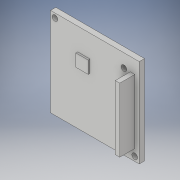
# Autodesk Inventor part: lab 04
Saved by Autodesk Inventor 2017 (Build 210142000, 142)
## iProperties
Created: 2016-10-26
Part Number: lab 04
Material: Generic
Document SubType Name: Modeling
Designer: radrajith
Density: 1 g/cm^3
Appearance: Default
Author: radrajith
Autodesk Inventor part; units mm, degrees
ref_plane "YZ Plane" through (0, 0, 0) normal (1, 0, 0) x (0, 1, 0)
ref_plane "XZ Plane" through (0, 0, 0) normal (0, 1, 0) x (-1, 0, 0)
ref_plane "XY Plane" through (0, 0, 0) normal (0, 0, 1) x (1, 0, 0)
sketch "Sketch1" plane through (0, 0, 0) normal (0, 0, 1) x (1, 0, 0)
  line L0 (0, 0) -> (50, 0)
  line L1 (50, 0) -> (50, 50)
  line L2 (50, 50) -> (0, 50)
  line L3 (0, 50) -> (0, 0)
  circle A0 centre (47.5, 2.5) radius 1.6
  circle A1 centre (41.39, 42.5) radius 1.6
  circle A2 centre (2.5, 47.5) radius 1.6
  dimension "d0" = 50
  dimension "d1" = 50
  dimension "d2" = 3.2
  dimension "d3" = 3.2
  dimension "d4" = 3.2
  constraints: 8 end point, 3 centre point, 2 parallel, 1 horizontal, 1 perpendicular
  measures "d0" distance of L2.end L1.end
  measures "d1" distance of L1.end L0.end
  measures "d2" diameter of A0
  measures "d3" diameter of A1
  measures "d4" diameter of A2
extrude "Extrusion1" add sketch "Sketch1" along normal blind 3
sketch "Sketch2" plane through (0, 0, 3) normal (0, 0, 1) x (1, 0, 0)
  line L0 (22.23, 30.37) -> (15.23, 30.37)
  line L1 (15.23, 30.37) -> (15.23, 37.37)
  line L2 (15.23, 37.37) -> (22.23, 37.37)
  line L3 (22.23, 37.37) -> (22.23, 30.37)
  point P0 (0, 0)
  dimension "d7" = 7
  dimension "d8" = 7
  constraints: 8 end point, 2 parallel, 1 horizontal, 1 perpendicular
  measures "d7" distance of L1.end L2.end
  measures "d8" distance of L0.end L1.end
extrude "Extrusion2" add sketch "Sketch2" along normal blind 1
sketch "Sketch3" plane through (0, 0, 3) normal (0, 0, 1) x (1, 0, 0)
  line L0 (47.541, 6.34) -> (45.001, 6.34)
  line L1 (45.001, 6.34) -> (45.001, 42.5)
  line L2 (45.001, 42.5) -> (47.541, 42.5)
  line L3 (47.541, 42.5) -> (47.541, 6.34)
  point P0 (0, 0)
  dimension "d11" = 2.54
  dimension "d12" = 36.16
  constraints: 8 end point, 2 parallel, 1 horizontal, 1 perpendicular
  measures "d11" distance of L1.end L2.end
  measures "d12" distance of L0.end L1.end
extrude "Extrusion3" add sketch "Sketch3" along normal blind 8.5
body "Solid1"
